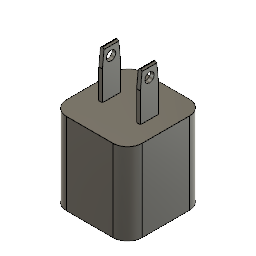
fu1 (Autodesk Fusion 360 design; units mm, degrees)
Autodesk Fusion 360 part; units mm, degrees
sketch "スケッチ1" plane through (0, 0, 0) normal (0, 1, 0) x (1, 0, 0)
  line L0 (-12.95, 13.1) -> (12.95, 13.1)
  line L1 (12.95, 13.1) -> (12.95, -13.1)
  line L2 (12.95, -13.1) -> (-12.95, -13.1)
  line L3 (-12.95, -13.1) -> (-12.95, 13.1)
  line L4 (5.85, 3.3) -> (5.85, -2.9)
  line L5 (5.85, -2.9) -> (5.85, 3.3)
  line L6 (7.15, -2.9) -> (7.15, 3.3)
  line L7 (5.85, 3.3) -> (7.15, 3.3)
  line L8 (7.15, -2.9) -> (5.85, -2.9)
  line L9 (-7.15, 3.3) -> (-5.85, 3.3)
  line L10 (-5.85, 3.3) -> (-5.85, -2.9)
  line L11 (-5.85, -2.9) -> (-7.15, -2.9)
  line L12 (-7.15, -2.9) -> (-7.15, 3.3)
  line L13 (-12.95, 13.1) -> (12.95, -13.1) construction
  dimension "d1" = 26.2
  dimension "d3" = 1.3
  dimension "d4" = 1.3
  dimension "d5" = 6.2
  dimension "d6" = 6.2
  dimension "d9" = 25.9
  dimension "d10" = 5.8
  dimension "d11" = 5.8
  dimension "d12" = 9.8
  dimension "d13" = 9.8
  measures "d1" distance of L0.end L1.end
  measures "d3" distance of L10 L12
  measures "d4" distance of L5 L6
  measures "d5" distance of L9.end L10.end
  measures "d6" distance of L6.end L6.start
  measures "d9" distance of L0.start L0.end
  measures "d10" distance of L3 L12
  measures "d11" distance of L1 L6
  measures "d12" distance of L0 L6.end
  measures "d13" distance of L0 L9.end
extrude "押し出し1" add sketch "スケッチ1" against normal blind 28 contours L0 L1 L2 L3 | L4 L5 L6 L7 L8 | L9 L10 L11 L12 makes body 1
extrude "押し出し2" add sketch "スケッチ1" along normal blind 16 contours L4 L5 L6 L7 L8 | L9 L10 L11 L12 bodies 1
fillet "フィレット1" radius 5 4 edges at (12.95, -14, 13.1) (-12.95, -14, 13.1) (12.95, -14, -13.1) (-12.95, -14, -13.1) on bodies 1
chamfer "面取り1" distance 0.6 distance2 6 4 edges at (-6.5, 16, -3.3) (-6.5, 16, 2.9) (6.5, 16, 2.9) (6.5, 16, -3.3) measured on face at (-6.7167, 16, -1.2333) measured on face at (-6.7167, 16, -1.2333) measured on face at (6.2833, 16, -1.2333) measured on face at (6.2833, 16, -1.2333) on bodies 1
chamfer "面取り2" distance 0.5 angle 45 4 edges at (-7.15, 16, -0.2) (-5.85, 16, -0.2) (5.85, 16, -0.2) (7.15, 16, -0.2) on bodies 1
hole "穴1" at (7.15, 12.4504, -0.2106) direction (-1, 0, 0) diameter 3.2 depth 6 tip angle 118 bodies 1
hole "穴2" at (-7.15, 12.5165, -0.0723) direction (1, 0, 0) diameter 3.2 depth 6 tip angle 118 bodies 1
sketch "スケッチ2" plane through (0, -28, 0) normal (0, -1, 0) x (1, 0, 0)
  arc A0 (-12.95, -8.1) -> (-7.95, -13.1) centre (-7.95, -8.1) ccw
  line L0 (-7.95, -13.1) -> (7.95, -13.1)
  arc A1 (7.95, -13.1) -> (12.95, -8.1) centre (7.95, -8.1) ccw
  line L1 (12.95, -8.1) -> (12.95, 8.1)
  arc A2 (12.95, 8.1) -> (7.95, 13.1) centre (7.95, 8.1) ccw
  line L2 (7.95, 13.1) -> (-7.95, 13.1)
  arc A3 (-7.95, 13.1) -> (-12.95, 8.1) centre (-7.95, 8.1) ccw
  line L3 (-12.95, 8.1) -> (-12.95, -8.1)
  line L4 (-6.75, 6.9) -> (5.95, 6.9)
  line L5 (5.95, 6.9) -> (5.95, 1.5)
  line L6 (5.95, 1.5) -> (-6.75, 1.5)
  line L7 (-6.75, 6.9) -> (-6.75, 1.5)
  line L8 (-5.85, 3.7624) -> (-5.85, 2.35)
  line L9 (-5.85, 2.35) -> (4.9348, 2.35)
  line L10 (4.9348, 2.35) -> (4.9348, 3.7624)
  line L11 (4.9348, 3.7624) -> (-5.85, 3.7624)
  dimension "d28" = 12.7
  dimension "d29" = 5.4
  dimension "d30" = 6.2
  dimension "d31" = 6.2
  measures "d28" distance of L4.start L4.end
  measures "d29" distance of L4.end L5.end
  measures "d30" distance of L2 L4
  measures "d31" distance of L3 L7
extrude "押し出し4" cut sketch "スケッチ2" against normal blind 3 contours L8 L9 L10 L11 bodies 1
extrude "押し出し3" cut sketch "スケッチ2" against normal blind 11.6 contours L4 L5 L6 L7 | L8 L9 L10 L11 bodies 1
extrude "押し出し5" add sketch "スケッチ2" against normal blind 11 separate body contours L8 L9 L10 L11 makes body 2
move_face "面をオフセット1" offset -3 1 faces at (1.3399, -28, 3.2916) on bodies 2
extrude "押し出し6" add 1 faces at (1.3399, -25, 3.2916) along direction (0, -1, 0) blind 1 on bodies 2 bodies 2
chamfer "面取り3" distance 0.25 angle 45 1 edges at (-0.4576, -26, 3.7624) on bodies 2
chamfer "面取り4" distance 0.25 angle 45 1 edges at (-0.4576, -26, 2.35) on bodies 2
chamfer "面取り5" distance 0.25 angle 45 1 edges at (4.9348, -26, 3.0562) on bodies 2
chamfer "面取り6" distance 0.25 angle 45 1 edges at (-5.85, -26, 3.0562) on bodies 2
sketch "スケッチ3" plane through (0, 0, 0) normal (1, 0, 0) x (0, 0, -1)
  line L0 (53.2263, 26.7652) -> (6.6913, 26.7652)
  line L1 (12.0596, -308.4214) -> (9.4485, 270.6965)
  line L2 (12.6899, -265.3742) -> (9.9887, 251.0729)
